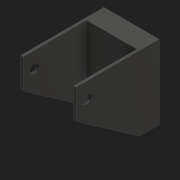
# Autodesk Inventor part: link_b2
Saved by Autodesk Inventor 2017 (Build 210142000, 142)
## iProperties
Created: 2019-08-03
Part Number: link_b2
Material: ABS Plastic
Document SubType Name: Modeling
Designer: Dell
Density: 1.06 g/cm^3
Appearance: Smooth - Black
Author: Dell
Autodesk Inventor part; units mm, degrees
ref_plane "YZ Plane" through (0, 0, 0) normal (1, 0, 0) x (0, 1, 0)
ref_plane "XZ Plane" through (0, 0, 0) normal (0, 1, 0) x (-1, 0, 0)
ref_plane "XY Plane" through (0, 0, 0) normal (0, 0, 1) x (1, 0, 0)
sketch "Sketch1" plane through (0, 0, 0) normal (0, 0, 1) x (1, 0, 0)
  line L0 (0, 0) -> (30, 0)
  line L1 (30, 0) -> (30, 45)
  line L2 (30, 45) -> (0, 45)
  line L3 (0, 45) -> (0, 0)
  dimension "d0" = 30
  dimension "d1" = 45
  constraints: 8 end point, 2 parallel, 1 horizontal, 1 perpendicular
  measures "d0" distance of L2.end L1.end
  measures "d1" distance of L1.end L0.end
extrude "Extrusion1" add sketch "Sketch1" along normal blind 40
sketch "Sketch2" plane through (0, 45, 0) normal (0, 1, 0) x (1, 0, 0)
  circle A0 centre (15, -17.7834) radius 7.5
  line L0 (30, -40) -> (0, -40) projected
  point P0 (0, 0)
  point P1 (15, -40)
  dimension "d4" = 15
  dimension "d5" = 22.2166
  constraints: 1 centre point, 1 midpoint, 1 vertical alignment
  measures "d4" diameter of A0
  measures "d5" distance from line of L0 A0.centre
extrude "Extrusion2" cut sketch "Sketch2" against normal blind 5
sketch "Sketch3" plane through (30, 0, 0) normal (1, 0, 0) x (0, 0, -1)
  circle A0 centre (-31.5856, 6) radius 2.5
  line L0 (0, 0) -> (-40, 0) projected
  line L1 (-40, 0) -> (-40, 45) projected
  dimension "d8" = 5
  dimension "d9" = 6
  dimension "d10" = 8.4144
  constraints: 1 centre point
  measures "d8" diameter of A0
  measures "d9" distance from line of L0 A0.centre
  measures "d10" distance from line of L1 A0.centre
extrude "Extrusion3" cut sketch "Sketch3" against normal through all
sketch "Sketch4" plane through (0, 0, 40) normal (0, 0, 1) x (1, 0, 0)
  line L0 (0, 45) -> (0, 0) projected
  line L1 (30, 0) -> (30, 45) projected
  line L2 (0, 0) -> (30, 0) projected
  line L3 (1.5, 0) -> (28.5, 0)
  line L4 (28.5, 0) -> (28.5, 34.2)
  line L5 (28.5, 34.2) -> (1.5, 34.2)
  line L6 (1.5, 34.2) -> (1.5, 0)
  point P0 (15, 0)
  dimension "d13" = 27
  dimension "d14" = 34.2
  constraints: 8 end point, 2 midpoint, 2 parallel, 1 horizontal, 1 perpendicular, 1 point on line
  measures "d13" distance of L4.end L5.end
  measures "d14" distance of L3.end L4.end
extrude "Extrusion4" cut sketch "Sketch4" against normal through all
sketch "Sketch5" plane through (30, 0, 0) normal (1, 0, 0) x (0, 0, -1)
  line L0 (-24, 0) -> (0, 34.2)
  line L1 (0, 0) -> (0, 45) projected
  line L2 (0, 0) -> (-40, 0) projected
  point P0 (-40, 34.2)
  dimension "d17" = 24
  constraints: 2 end point, 2 point on line, 1 horizontal alignment
  measures "d17" horizontal distance of L0.end L0.start
extrude "Extrusion5" cut sketch "Sketch5" against normal through all
body "Solid1"
